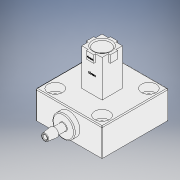
# Autodesk Inventor part: 9mm_ball_holder
Saved by Autodesk Inventor 2019 (Build 230136000, 136)
## iProperties
Created: 2019-03-11
Part Number: 9mm_ball_holder
Material: ABS Plastic
Document SubType Name: Modeling
Designer: Wilson Lab
Density: 1.06 g/cm^3
Appearance: Smooth - White
Author: Wilson Lab
Autodesk Inventor part; units mm, degrees
ref_plane "YZ Plane" through (0, 0, 0) normal (1, 0, 0) x (0, 1, 0)
ref_plane "XZ Plane" through (0, 0, 0) normal (0, 1, 0) x (-1, 0, 0)
ref_plane "XY Plane" through (0, 0, 0) normal (0, 0, 1) x (1, 0, 0)
sketch "Sketch1" plane through (0, 0, 0) normal (0, 0, 1) x (1, 0, 0)
  line L0 (0, 0) -> (-5.5, 0) construction
  line L1 (-5.5, 0) -> (-5.5, 20) construction
  line L2 (-5.5, 20) -> (0, 20) construction
  line L3 (0, 20) -> (0, 0) construction
  circle A0 centre (0, 20.35) radius 4.5 construction
  line L4 (-5.5, 20) -> (-5.1335, 20)
  line L5 (-0.75, 15.3188) -> (-0.75, 0)
  arc A1 (-4.4001, 19.4071) -> (-1.2857, 16.0376) centre (0, 20.35) ccw
  arc A2 (-0.75, 15.3188) -> (-1.2857, 16.0376) centre (-1.5, 15.3188) ccw
  arc A3 (-4.4001, 19.4071) -> (-5.1335, 20) centre (-5.1335, 19.25) ccw
  line L6 (-5.5, 20) -> (-5.5, 0)
  line L7 (-5.5, 0) -> (-0.75, 0)
  point P0 (-4.4864, 20)
  point P1 (-0.75, 15.9129)
  dimension "d1" = 20
  dimension "d5" = 9
  dimension "d6" = 0.35
  dimension "d7" = 0.75
  dimension "d8" = 0.75
  dimension "d9" = 0.75
  dimension "d133" = 5.5
  dimension "d134" = 1.0136
  constraints: 18 end point, 10 point on circle, 5 point on line, 4 centre point, 4 tangent, 3 perpendicular, 2 parallel, 1 collinear, 1 concentric, 1 horizontal
  measures "d1" distance between parallel lines of L0 L2
  measures "d5" diameter of A0
  measures "d6" distance of A0.centre L2.end
  measures "d7" distance between parallel lines of L3 L5
  measures "d8" radius of A2
  measures "d9" radius of A3
  measures "d133" distance between parallel lines of L1 L3
  measures "d134" distance of A0.start L1.end
revolve "Revolution1" add sketch "Sketch1" angle 360 about axis through (0, 20, 0) along (0, -1, 0)
ref_plane "Work Plane1" through (0, 20, 0) normal (0, 1, 0) x (1, 0, 0)
sketch "Sketch2" plane through (0, 20, 0) normal (0, 1, 0) x (1, 0, 0)
  circle A0 centre (0, 0) radius 5.5 projected
  circle A1 centre (0, 0) radius 5.5 construction
  line L0 (-5.5, -5.5) -> (5.5, -5.5)
  line L1 (5.5, -5.5) -> (5.5, 5.5)
  line L2 (5.5, 5.5) -> (-5.5, 5.5)
  line L3 (-5.5, 5.5) -> (-5.5, -5.5)
  circle A2 centre (0, 0) radius 1.2857 projected
  line L4 (-5.5, -5.5) -> (5.5, 5.5) construction
  line L5 (5.5, -5.5) -> (-5.5, 5.5) construction
  point P0 (0, 0)
  dimension "d124" = 0
  constraints: 12 end point, 2 midpoint, 2 parallel, 2 tangent, 1 centre point, 1 coincident, 1 horizontal, 1 perpendicular
  measures "d124" distance edge to line of A0 L1
extrude "Extrusion1" add sketch "Sketch2" against normal up to surface (20 mm away) contours L1 L0 A0 | A0 L2 L1 | A0 L3 L2 | L0 L3 A0
ref_plane "Work Plane7" through (0, 0, 0) normal (0, -1, 0) x (1, 0, 0)
sketch "Sketch11" plane through (0, 0, 0) normal (0, -1, 0) x (1, 0, 0)
  line L0 (0, 18) -> (0, 0) construction
  line L1 (-18, -18) -> (18, -18)
  line L2 (18, -18) -> (18, 18)
  line L3 (18, 18) -> (-18, 18)
  line L4 (-18, 18) -> (-18, -18)
  line L5 (-18, -18) -> (18, 18) construction
  line L6 (18, -18) -> (-18, 18) construction
  dimension "d60" = 36
  dimension "d61" = 36
  constraints: 14 end point, 3 midpoint, 2 parallel, 1 horizontal, 1 perpendicular
  measures "d60" distance of L1.end L2.end
  measures "d61" distance of L2.end L3.end
extrude "Extrusion6" add sketch "Sketch11" along normal blind 15
sketch "Sketch16" plane through (-18, 0, -18) normal (-1, 0, 0) x (0, 0, 1)
  line L0 (36, 0) -> (0, 0) construction
  line L1 (0, 0) -> (0, -15) construction
  line L2 (36, -15) -> (0, -15) construction
  line L3 (36, 0) -> (36, -15) construction
  line L4 (18.75, 15.3188) -> (18.75, 0) construction
  line L5 (17.25, 15.3188) -> (17.25, 0) construction
  line L6 (18, -7.5) -> (18, 0) construction
  line L7 (36, 0) -> (36, -15) construction
  line L8 (36, 0) -> (36, -7.5) construction
  line L9 (18, -7.5) -> (36, -7.5) construction
  circle A0 centre (18, -7.5) radius 4.225
  dimension "d64" = 8.45
  constraints: 6 end point, 1 centre point, 1 coincident, 1 horizontal, 1 midpoint, 1 vertical
  measures "d64" diameter of A0
extrude "Extrusion7" cut sketch "Sketch16" against normal blind 32.7
sketch "Sketch17" plane through (0, 0, 0) normal (0, -1, 0) x (1, 0, 0)
  circle A0 centre (0, 0) radius 0.75 projected
  point P0 (0, 0)
ref_plane "Work Plane8" through (-18, 0, 0) normal (0, 0, 1) x (1, 0, 0)
sketch "Sketch18" plane through (-18, 0, 0) normal (0, 0, 1) x (1, 0, 0)
  line L0 (18, 0) -> (18, -10.576)
  line L1 (0, -11.725) -> (32.7, -11.725) projected
  constraints: 2 end point, 1 vertical
sweep "Sweep3" cut profiles "Sketch17" path "Sketch18" path curves L0
fillet "Fillet1" radius 3 1 edges at (-0.75, -3.275, -0.001)
sketch "Sketch19" plane through (0, 0, 0) normal (0, 1, 0) x (1, 0, 0)
  line L0 (18, -18) -> (-18, -18) construction
  line L1 (18, 18) -> (18, -18) construction
  line L2 (-18, 18) -> (18, 18) construction
  line L3 (-18, -18) -> (-18, 18) construction
  line L4 (-12.7, 12.7) -> (12.7, 12.7) construction
  line L5 (12.7, 12.7) -> (12.7, -12.7) construction
  line L6 (12.7, -12.7) -> (-12.7, -12.7) construction
  line L7 (-12.7, -12.7) -> (-12.7, 12.7) construction
  circle A0 centre (0, 0) radius 1.2857 construction
  line L8 (-12.7, 12.7) -> (12.7, -12.7) construction
  line L9 (12.7, 12.7) -> (-12.7, -12.7) construction
  point P0 (0, 0)
  dimension "d70" = 25.4
  dimension "d71" = 25.4
  constraints: 12 end point, 4 coincident, 2 midpoint, 2 parallel, 1 horizontal, 1 perpendicular
  measures "d70" distance of L4.end L5.end
  measures "d71" distance of L5.end L6.end
hole "Hole3" at (12.7, 0, -12.7) at (12.7, 0, 12.7) at (-12.7, 0, 12.7) at (-12.7, 0, -12.7) direction (0, -1, 0) diameter 4.496 end through all counterbore diameter 7.938 counterbore depth 4.166
sketch "Sketch21" plane through (-18, 0, 0) normal (0, 0, 1) x (1, 0, 0)
  line L0 (0, -11.725) -> (0, -3.275) construction
  line L1 (0, 0) -> (0, -15) construction
  line L2 (0, -7.5) -> (-3, -7.5)
  line L3 (-3, -9.6296) -> (-3, -13.5)
  line L4 (-3, -13.5) -> (0, -13.5)
  line L5 (0, -13.5) -> (0, -7.5) construction
  line L6 (-3.25, -9.3796) -> (-8, -9.3796)
  arc A0 (-3, -9.6296) -> (-3.25, -9.3796) centre (-3.25, -9.6296) ccw
  line L7 (-8, -9.3796) -> (-8, -9.913)
  line L8 (-8, -9.913) -> (-12.8561, -9.4031)
  line L9 (-8, -9.3796) -> (-13.08, -9.3796) construction
  line L10 (-12.83, -8.65) -> (0, -8.65)
  line L11 (-13.08, -8.9) -> (-13.08, -9.1545)
  arc A1 (-12.83, -8.65) -> (-13.08, -8.9) centre (-12.83, -8.9) ccw
  arc A2 (-13.08, -9.1545) -> (-12.8561, -9.4031) centre (-12.83, -9.1545) ccw
  line L12 (0, -8.65) -> (0, -13.5)
  point P0 (18, 0)
  point P1 (-3, -9.3796)
  dimension "d79" = 3
  dimension "d80" = 6
  dimension "d81" = 5
  dimension "d82" = 1.8796
  dimension "d83" = 0.25
  dimension "d84" = 2.413
  dimension "d85" = 5.08
  dimension "d86" = 1.15
  dimension "d87" = 0.25
  dimension "d88" = 0.25
  constraints: 22 end point, 6 point on circle, 6 point on line, 6 tangent, 3 centre point, 3 horizontal, 2 parallel, 2 perpendicular, 2 vertical, 1 collinear, 1 midpoint
  measures "d79" distance of L3.end L4.end
  measures "d80" distance between parallel lines of L2 L4
  measures "d81" distance of point (-3, -9.38) L6.end
  measures "d82" distance between parallel lines of L2 L6
  measures "d83" radius of A0
  measures "d84" distance from line of L2 L7.end
  measures "d85" horizontal distance of L7.end L9.end
  measures "d86" distance between parallel lines of L10 L2
  measures "d87" radius of A1
  measures "d88" radius of A2
revolve "Revolution2" add sketch "Sketch21" angle 360 about axis through (-18, -7.5, 0) along (-1, 0, 0)
fillet "Fillet2" radius 0.5 9 edges at (-21, -1.5, 0) (0, 0, -18) (-18, 0, 0) (0, 0, 18) (18, 0, 0) (18, -7.5, 18) (-18, -7.5, 18) (-18, -7.5, -18) (18, -7.5, -18)
sketch "Sketch28" plane through (-5.5, 20, -5.5) normal (-1, 0, 0) x (0, 0, 1)
  line L0 (0, -20) -> (11, -20) construction
  line L1 (11, 0) -> (11, -20) construction
  line L2 (0, 0) -> (11, 0) construction
  line L3 (0, 0) -> (0, -20) construction
  line L4 (3.5, -4) -> (7.5, -4)
  line L5 (7.5, -4) -> (7.5, 0)
  line L6 (7.5, 0) -> (3.5, 0)
  line L7 (3.5, 0) -> (3.5, -4)
  line L8 (3.5, -2) -> (0, -2) construction
  line L9 (7.5, -2) -> (11, -2) construction
  point P0 (5.5, -20)
  dimension "d125" = 0
  dimension "d126" = 4
  constraints: 12 end point, 3 point on line, 2 equal length, 2 midpoint, 2 parallel, 2 perpendicular, 1 horizontal
  measures "d125" distance between parallel lines of L2 L6
  measures "d126" distance of L4.end L5.end
extrude "Extrusion13" add sketch "Sketch28" along normal blind 1
pattern_circular "Circular Pattern1" count 4 over 360 about axis through (0, -10, 0) along (0, 1, 0) of "Extrusion13"
sketch "Sketch29" plane through (-5.5, 0, -5.5) normal (-1, 0, 0) x (0, 0, 1)
  line L0 (0, 20) -> (0, 0) construction
  line L1 (0, 10) -> (11, 10) construction
  line L2 (11, 20) -> (11, 0) construction
  line L3 (0, 10) -> (11, 10) construction
  line L4 (11, 10) -> (11, 8) construction
  line L5 (11, 8) -> (0, 8) construction
  line L6 (0, 8) -> (0, 10) construction
  line L7 (0, 9) -> (11, 9) construction
  line L8 (11, 20) -> (11, 0) construction
  line L9 (0, 10) -> (0, 9) construction
  line L10 (11, 10) -> (11, 9) construction
  spline S0 degree 2 poles (4.1469, 9.0742) (4.1469, 9.0526) (4.1423, 9.0225) (4.1338, 9.0047) (4.1235, 8.9972) (4.116, 8.9972) knots 0 0 0 1 2 3 4 4 4
  line L11 (4.116, 8.9972) -> (3.5667, 8.9972)
  spline S1 degree 2 poles (3.5667, 8.9972) (3.5601, 8.9972) (3.5498, 9.0047) (3.5413, 9.0225) (3.5366, 9.0526) (3.5366, 9.0742) knots 0 0 0 1 2 3 4 4 4
  spline S2 degree 2 poles (3.5366, 9.0742) (3.5366, 9.0958) (3.5404, 9.1258) (3.5488, 9.1446) (3.5601, 9.1531) (3.5667, 9.1531) knots 0 0 0 1 2 3 4 4 4
  line L12 (3.5667, 9.1531) -> (3.7516, 9.1531)
  line L13 (3.7516, 9.1531) -> (3.7516, 9.8019)
  line L14 (3.7516, 9.8019) -> (3.5911, 9.7136)
  spline S3 degree 2 poles (3.5911, 9.7136) (3.5742, 9.7052) (3.5516, 9.7014) (3.5385, 9.7146) (3.5338, 9.7465) (3.5338, 9.7756) knots 0 0 0 1 2 3 4 4 4
  spline S4 degree 2 poles (3.5338, 9.7756) (3.5338, 9.7944) (3.5357, 9.8178) (3.5413, 9.8347) (3.5526, 9.846) (3.562, 9.8516) knots 0 0 0 1 2 3 4 4 4
  line L15 (3.562, 9.8516) -> (3.7751, 9.9897)
  spline S5 degree 2 poles (3.7751, 9.9897) (3.7798, 9.9934) (3.7911, 9.9972) (3.8099, 9.9991) (3.8399, 10) (3.8634, 10) knots 0 0 0 1 2 3 4 4 4
  spline S6 degree 2 poles (3.8634, 10) (3.8925, 10) (3.9291, 9.9981) (3.9469, 9.9925) (3.9535, 9.9831) (3.9535, 9.9765) knots 0 0 0 1 2 3 4 4 4
  line L16 (3.9535, 9.9765) -> (3.9535, 9.1531)
  line L17 (3.9535, 9.1531) -> (4.116, 9.1531)
  spline S7 degree 2 poles (4.116, 9.1531) (4.1235, 9.1531) (4.1347, 9.1446) (4.1432, 9.1258) (4.1469, 9.0958) (4.1469, 9.0742) knots 0 0 0 1 2 3 4 4 4
  spline S8 degree 2 poles (4.9451, 9.0742) (4.9451, 9.0526) (4.9404, 9.0225) (4.9319, 9.0047) (4.9216, 8.9972) (4.9141, 8.9972) knots 0 0 0 1 2 3 4 4 4
  line L18 (4.9141, 8.9972) -> (4.3648, 8.9972)
  spline S9 degree 2 poles (4.3648, 8.9972) (4.3582, 8.9972) (4.3479, 9.0047) (4.3394, 9.0225) (4.3347, 9.0526) (4.3347, 9.0742) knots 0 0 0 1 2 3 4 4 4
  spline S10 degree 2 poles (4.3347, 9.0742) (4.3347, 9.0958) (4.3385, 9.1258) (4.3469, 9.1446) (4.3582, 9.1531) (4.3648, 9.1531) knots 0 0 0 1 2 3 4 4 4
  line L19 (4.3648, 9.1531) -> (4.5498, 9.1531)
  line L20 (4.5498, 9.1531) -> (4.5498, 9.8019)
  line L21 (4.5498, 9.8019) -> (4.3892, 9.7136)
  spline S11 degree 2 poles (4.3892, 9.7136) (4.3723, 9.7052) (4.3498, 9.7014) (4.3366, 9.7146) (4.3319, 9.7465) (4.3319, 9.7756) knots 0 0 0 1 2 3 4 4 4
  spline S12 degree 2 poles (4.3319, 9.7756) (4.3319, 9.7944) (4.3338, 9.8178) (4.3394, 9.8347) (4.3507, 9.846) (4.3601, 9.8516) knots 0 0 0 1 2 3 4 4 4
  line L22 (4.3601, 9.8516) -> (4.5732, 9.9897)
  spline S13 degree 2 poles (4.5732, 9.9897) (4.5779, 9.9934) (4.5892, 9.9972) (4.608, 9.9991) (4.638, 10) (4.6615, 10) knots 0 0 0 1 2 3 4 4 4
  spline S14 degree 2 poles (4.6615, 10) (4.6906, 10) (4.7272, 9.9981) (4.7451, 9.9925) (4.7516, 9.9831) (4.7516, 9.9765) knots 0 0 0 1 2 3 4 4 4
  line L23 (4.7516, 9.9765) -> (4.7516, 9.1531)
  line L24 (4.7516, 9.1531) -> (4.9141, 9.1531)
  spline S15 degree 2 poles (4.9141, 9.1531) (4.9216, 9.1531) (4.9329, 9.1446) (4.9413, 9.1258) (4.9451, 9.0958) (4.9451, 9.0742) knots 0 0 0 1 2 3 4 4 4
  spline S16 degree 2 poles (6.2052, 9.0235) (6.2052, 9.016) (6.1958, 9.0038) (6.1742, 8.9962) (6.1376, 8.9925) (6.1085, 8.9925) knots 0 0 0 1 2 3 4 4 4
  spline S17 degree 2 poles (6.1085, 8.9925) (6.0793, 8.9925) (6.0427, 8.9962) (6.0202, 9.0038) (6.0117, 9.016) (6.0117, 9.0235) knots 0 0 0 1 2 3 4 4 4
  line L25 (6.0117, 9.0235) -> (6.0117, 9.43)
  spline S18 degree 2 poles (6.0117, 9.43) (6.0117, 9.4648) (5.9986, 9.5221) (5.9723, 9.5624) (5.931, 9.585) (5.9028, 9.585) knots 0 0 0 1 2 3 4 4 4
  spline S19 degree 2 poles (5.9028, 9.585) (5.8681, 9.585) (5.7977, 9.5315) (5.7563, 9.4798) knots 0 0 0 1 2 2 2
  line L26 (5.7563, 9.4798) -> (5.7563, 9.0235)
  spline S20 degree 2 poles (5.7563, 9.0235) (5.7563, 9.016) (5.7469, 9.0038) (5.7244, 8.9962) (5.6878, 8.9925) (5.6596, 8.9925) knots 0 0 0 1 2 3 4 4 4
  spline S21 degree 2 poles (5.6596, 8.9925) (5.6315, 8.9925) (5.5948, 8.9962) (5.5723, 9.0038) (5.5629, 9.016) (5.5629, 9.0235) knots 0 0 0 1 2 3 4 4 4
  line L27 (5.5629, 9.0235) -> (5.5629, 9.43)
  spline S22 degree 2 poles (5.5629, 9.43) (5.5629, 9.4648) (5.5498, 9.5221) (5.5235, 9.5624) (5.4822, 9.585) (5.454, 9.585) knots 0 0 0 1 2 3 4 4 4
  spline S23 degree 2 poles (5.454, 9.585) (5.4183, 9.585) (5.3479, 9.5315) (5.3066, 9.4798) knots 0 0 0 1 2 2 2
  line L28 (5.3066, 9.4798) -> (5.3066, 9.0235)
  spline S24 degree 2 poles (5.3066, 9.0235) (5.3066, 9.016) (5.2972, 9.0038) (5.2746, 8.9962) (5.238, 8.9925) (5.2099, 8.9925) knots 0 0 0 1 2 3 4 4 4
  spline S25 degree 2 poles (5.2099, 8.9925) (5.1817, 8.9925) (5.1451, 8.9962) (5.1225, 9.0038) (5.1131, 9.016) (5.1131, 9.0235) knots 0 0 0 1 2 3 4 4 4
  line L29 (5.1131, 9.0235) -> (5.1131, 9.7089)
  spline S26 degree 2 poles (5.1131, 9.7089) (5.1131, 9.7164) (5.1207, 9.7286) (5.1404, 9.7362) (5.1723, 9.7399) (5.1958, 9.7399) knots 0 0 0 1 2 3 4 4 4
  spline S27 degree 2 poles (5.1958, 9.7399) (5.2202, 9.7399) (5.2531, 9.7362) (5.2709, 9.7286) (5.2784, 9.7164) (5.2784, 9.7089) knots 0 0 0 1 2 3 4 4 4
  line L30 (5.2784, 9.7089) -> (5.2784, 9.63)
  spline S28 degree 2 poles (5.2784, 9.63) (5.3357, 9.6911) (5.4484, 9.7531) (5.5103, 9.7531) knots 0 0 0 1 2 2 2
  spline S29 degree 2 poles (5.5103, 9.7531) (5.5526, 9.7531) (5.6202, 9.7352) (5.6737, 9.7023) (5.7122, 9.6563) (5.7254, 9.6272) knots 0 0 0 1 2 3 4 4 4
  spline S30 degree 2 poles (5.7254, 9.6272) (5.7563, 9.661) (5.8155, 9.708) (5.8728, 9.738) (5.931, 9.7531) (5.961, 9.7531) knots 0 0 0 1 2 3 4 4 4
  spline S31 degree 2 poles (5.961, 9.7531) (6.0296, 9.7531) (6.1225, 9.707) (6.1808, 9.6282) (6.2052, 9.5211) (6.2052, 9.462) knots 0 0 0 1 2 3 4 4 4
  line L31 (6.2052, 9.462) -> (6.2052, 9.0235)
  spline S32 degree 2 poles (7.4869, 9.0235) (7.4869, 9.016) (7.4775, 9.0038) (7.4559, 8.9962) (7.4192, 8.9925) (7.3901, 8.9925) knots 0 0 0 1 2 3 4 4 4
  spline S33 degree 2 poles (7.3901, 8.9925) (7.361, 8.9925) (7.3244, 8.9962) (7.3019, 9.0038) (7.2934, 9.016) (7.2934, 9.0235) knots 0 0 0 1 2 3 4 4 4
  line L32 (7.2934, 9.0235) -> (7.2934, 9.43)
  spline S34 degree 2 poles (7.2934, 9.43) (7.2934, 9.4648) (7.2803, 9.5221) (7.254, 9.5624) (7.2127, 9.585) (7.1845, 9.585) knots 0 0 0 1 2 3 4 4 4
  spline S35 degree 2 poles (7.1845, 9.585) (7.1498, 9.585) (7.0793, 9.5315) (7.038, 9.4798) knots 0 0 0 1 2 2 2
  line L33 (7.038, 9.4798) -> (7.038, 9.0235)
  spline S36 degree 2 poles (7.038, 9.0235) (7.038, 9.016) (7.0286, 9.0038) (7.0061, 8.9962) (6.9695, 8.9925) (6.9413, 8.9925) knots 0 0 0 1 2 3 4 4 4
  spline S37 degree 2 poles (6.9413, 8.9925) (6.9131, 8.9925) (6.8765, 8.9962) (6.854, 9.0038) (6.8446, 9.016) (6.8446, 9.0235) knots 0 0 0 1 2 3 4 4 4
  line L34 (6.8446, 9.0235) -> (6.8446, 9.43)
  spline S38 degree 2 poles (6.8446, 9.43) (6.8446, 9.4648) (6.8315, 9.5221) (6.8052, 9.5624) (6.7638, 9.585) (6.7357, 9.585) knots 0 0 0 1 2 3 4 4 4
  spline S39 degree 2 poles (6.7357, 9.585) (6.7, 9.585) (6.6296, 9.5315) (6.5883, 9.4798) knots 0 0 0 1 2 2 2
  line L35 (6.5883, 9.4798) -> (6.5883, 9.0235)
  spline S40 degree 2 poles (6.5883, 9.0235) (6.5883, 9.016) (6.5789, 9.0038) (6.5563, 8.9962) (6.5197, 8.9925) (6.4915, 8.9925) knots 0 0 0 1 2 3 4 4 4
  spline S41 degree 2 poles (6.4915, 8.9925) (6.4634, 8.9925) (6.4268, 8.9962) (6.4042, 9.0038) (6.3948, 9.016) (6.3948, 9.0235) knots 0 0 0 1 2 3 4 4 4
  line L36 (6.3948, 9.0235) -> (6.3948, 9.7089)
  spline S42 degree 2 poles (6.3948, 9.7089) (6.3948, 9.7164) (6.4023, 9.7286) (6.4221, 9.7362) (6.454, 9.7399) (6.4775, 9.7399) knots 0 0 0 1 2 3 4 4 4
  spline S43 degree 2 poles (6.4775, 9.7399) (6.5019, 9.7399) (6.5347, 9.7362) (6.5526, 9.7286) (6.5601, 9.7164) (6.5601, 9.7089) knots 0 0 0 1 2 3 4 4 4
  line L37 (6.5601, 9.7089) -> (6.5601, 9.63)
  spline S44 degree 2 poles (6.5601, 9.63) (6.6174, 9.6911) (6.73, 9.7531) (6.792, 9.7531) knots 0 0 0 1 2 2 2
  spline S45 degree 2 poles (6.792, 9.7531) (6.8343, 9.7531) (6.9019, 9.7352) (6.9554, 9.7023) (6.9939, 9.6563) (7.007, 9.6272) knots 0 0 0 1 2 3 4 4 4
  spline S46 degree 2 poles (7.007, 9.6272) (7.038, 9.661) (7.0972, 9.708) (7.1545, 9.738) (7.2127, 9.7531) (7.2427, 9.7531) knots 0 0 0 1 2 3 4 4 4
  spline S47 degree 2 poles (7.2427, 9.7531) (7.3113, 9.7531) (7.4042, 9.707) (7.4624, 9.6282) (7.4869, 9.5211) (7.4869, 9.462) knots 0 0 0 1 2 3 4 4 4
  line L38 (7.4869, 9.462) -> (7.4869, 9.0235)
  point P0 (5.5, 0)
  dimension "d139" = 1
  constraints: 8 end point, 5 midpoint, 2 coincident, 2 collinear, 1 horizontal, 1 point on line, 2 other
  measures "d139" distance between parallel lines of L7 L1
sketch "Sketch30" plane through (-6.5, 20, -5.5) normal (-1, 0, 0) x (0, 0, 1)
  line L0 (3.5, 0) -> (3.5, -4) construction
  line L1 (3.5, -2) -> (7.5, -2) construction
  line L2 (7.5, 0) -> (7.5, -4) construction
  line L3 (3.5, -2) -> (7.5, -2) construction
  line L4 (7.5, -2) -> (7.5, -5.2981) construction
  line L5 (7.5, -5.2981) -> (3.5, -5.2981) construction
  line L6 (3.5, -5.2981) -> (3.5, -2) construction
  line L7 (7.5, -4) -> (7.5, 0) projected
  spline S0 degree 2 poles (4.5864, -2.7146) (4.5864, -2.754) (4.5704, -2.7944) (4.5563, -2.7944) knots 0 0 0 1 2 2 2
  line L8 (4.5563, -2.7944) -> (4.4681, -2.7944)
  line L9 (4.4681, -2.7944) -> (4.4681, -2.9737)
  spline S1 degree 2 poles (4.4681, -2.9737) (4.4681, -2.9812) (4.4587, -2.9934) (4.4362, -3.0009) (4.3986, -3.0047) (4.3695, -3.0047) knots 0 0 0 1 2 3 4 4 4
  spline S2 degree 2 poles (4.3695, -3.0047) (4.3423, -3.0047) (4.3047, -3.0009) (4.2822, -2.9934) (4.2737, -2.9812) (4.2737, -2.9737) knots 0 0 0 1 2 3 4 4 4
  line L10 (4.2737, -2.9737) -> (4.2737, -2.7944)
  line L11 (4.2737, -2.7944) -> (3.8925, -2.7944)
  spline S3 degree 2 poles (3.8925, -2.7944) (3.8812, -2.7944) (3.8643, -2.7887) (3.8531, -2.77) (3.8474, -2.7333) (3.8474, -2.7033) knots 0 0 0 1 2 3 4 4 4
  spline S4 degree 2 poles (3.8474, -2.7033) (3.8474, -2.6789) (3.8493, -2.6432) (3.8549, -2.6131) (3.8653, -2.5878) (3.8728, -2.5728) knots 0 0 0 1 2 3 4 4 4
  line L12 (3.8728, -2.5728) -> (4.1826, -2.0272)
  spline S5 degree 2 poles (4.1826, -2.0272) (4.1864, -2.0197) (4.2052, -2.0103) (4.238, -2.0028) (4.2887, -2) (4.3254, -2) knots 0 0 0 1 2 3 4 4 4
  spline S6 degree 2 poles (4.3254, -2) (4.3648, -2) (4.4192, -2.0038) (4.4531, -2.0122) (4.4681, -2.0244) (4.4681, -2.0329) knots 0 0 0 1 2 3 4 4 4
  line L13 (4.4681, -2.0329) -> (4.4681, -2.6329)
  line L14 (4.4681, -2.6329) -> (4.5563, -2.6329)
  spline S7 degree 2 poles (4.5563, -2.6329) (4.5685, -2.6329) (4.5864, -2.6704) (4.5864, -2.7146) knots 0 0 0 1 2 2 2
  line L15 (4.2737, -2.1746) -> (4.2718, -2.1746)
  line L16 (4.2718, -2.1746) -> (4.0089, -2.6329)
  line L17 (4.0089, -2.6329) -> (4.2737, -2.6329)
  line L18 (4.2737, -2.6329) -> (4.2737, -2.1746)
  spline S8 degree 2 poles (5.8061, -2.9737) (5.8061, -2.9812) (5.7967, -2.9934) (5.7751, -3.0009) (5.7385, -3.0047) (5.7094, -3.0047) knots 0 0 0 1 2 3 4 4 4
  spline S9 degree 2 poles (5.7094, -3.0047) (5.6803, -3.0047) (5.6437, -3.0009) (5.6211, -2.9934) (5.6127, -2.9812) (5.6127, -2.9737) knots 0 0 0 1 2 3 4 4 4
  line L19 (5.6127, -2.9737) -> (5.6127, -2.5671)
  spline S10 degree 2 poles (5.6127, -2.5671) (5.6127, -2.5324) (5.5995, -2.4751) (5.5732, -2.4347) (5.5319, -2.4122) (5.5038, -2.4122) knots 0 0 0 1 2 3 4 4 4
  spline S11 degree 2 poles (5.5038, -2.4122) (5.469, -2.4122) (5.3986, -2.4657) (5.3573, -2.5174) knots 0 0 0 1 2 2 2
  line L20 (5.3573, -2.5174) -> (5.3573, -2.9737)
  spline S12 degree 2 poles (5.3573, -2.9737) (5.3573, -2.9812) (5.3479, -2.9934) (5.3254, -3.0009) (5.2887, -3.0047) (5.2606, -3.0047) knots 0 0 0 1 2 3 4 4 4
  spline S13 degree 2 poles (5.2606, -3.0047) (5.2324, -3.0047) (5.1958, -3.0009) (5.1732, -2.9934) (5.1638, -2.9812) (5.1638, -2.9737) knots 0 0 0 1 2 3 4 4 4
  line L21 (5.1638, -2.9737) -> (5.1638, -2.5671)
  spline S14 degree 2 poles (5.1638, -2.5671) (5.1638, -2.5324) (5.1507, -2.4751) (5.1244, -2.4347) (5.0831, -2.4122) (5.0549, -2.4122) knots 0 0 0 1 2 3 4 4 4
  spline S15 degree 2 poles (5.0549, -2.4122) (5.0192, -2.4122) (4.9488, -2.4657) (4.9075, -2.5174) knots 0 0 0 1 2 2 2
  line L22 (4.9075, -2.5174) -> (4.9075, -2.9737)
  spline S16 degree 2 poles (4.9075, -2.9737) (4.9075, -2.9812) (4.8981, -2.9934) (4.8756, -3.0009) (4.839, -3.0047) (4.8108, -3.0047) knots 0 0 0 1 2 3 4 4 4
  spline S17 degree 2 poles (4.8108, -3.0047) (4.7826, -3.0047) (4.746, -3.0009) (4.7235, -2.9934) (4.7141, -2.9812) (4.7141, -2.9737) knots 0 0 0 1 2 3 4 4 4
  line L23 (4.7141, -2.9737) -> (4.7141, -2.2883)
  spline S18 degree 2 poles (4.7141, -2.2883) (4.7141, -2.2808) (4.7216, -2.2685) (4.7413, -2.261) (4.7732, -2.2573) (4.7967, -2.2573) knots 0 0 0 1 2 3 4 4 4
  spline S19 degree 2 poles (4.7967, -2.2573) (4.8211, -2.2573) (4.854, -2.261) (4.8718, -2.2685) (4.8793, -2.2808) (4.8793, -2.2883) knots 0 0 0 1 2 3 4 4 4
  line L24 (4.8793, -2.2883) -> (4.8793, -2.3671)
  spline S20 degree 2 poles (4.8793, -2.3671) (4.9366, -2.3061) (5.0493, -2.2441) (5.1113, -2.2441) knots 0 0 0 1 2 2 2
  spline S21 degree 2 poles (5.1113, -2.2441) (5.1535, -2.2441) (5.2211, -2.262) (5.2746, -2.2948) (5.3131, -2.3408) (5.3263, -2.37) knots 0 0 0 1 2 3 4 4 4
  spline S22 degree 2 poles (5.3263, -2.37) (5.3573, -2.3362) (5.4164, -2.2892) (5.4737, -2.2592) (5.5319, -2.2441) (5.562, -2.2441) knots 0 0 0 1 2 3 4 4 4
  spline S23 degree 2 poles (5.562, -2.2441) (5.6305, -2.2441) (5.7235, -2.2901) (5.7817, -2.369) (5.8061, -2.4761) (5.8061, -2.5352) knots 0 0 0 1 2 3 4 4 4
  line L25 (5.8061, -2.5352) -> (5.8061, -2.9737)
  spline S24 degree 2 poles (7.0878, -2.9737) (7.0878, -2.9812) (7.0784, -2.9934) (7.0568, -3.0009) (7.0202, -3.0047) (6.9911, -3.0047) knots 0 0 0 1 2 3 4 4 4
  spline S25 degree 2 poles (6.9911, -3.0047) (6.962, -3.0047) (6.9254, -3.0009) (6.9028, -2.9934) (6.8944, -2.9812) (6.8944, -2.9737) knots 0 0 0 1 2 3 4 4 4
  line L26 (6.8944, -2.9737) -> (6.8944, -2.5671)
  spline S26 degree 2 poles (6.8944, -2.5671) (6.8944, -2.5324) (6.8812, -2.4751) (6.8549, -2.4347) (6.8136, -2.4122) (6.7854, -2.4122) knots 0 0 0 1 2 3 4 4 4
  spline S27 degree 2 poles (6.7854, -2.4122) (6.7507, -2.4122) (6.6803, -2.4657) (6.639, -2.5174) knots 0 0 0 1 2 2 2
  line L27 (6.639, -2.5174) -> (6.639, -2.9737)
  spline S28 degree 2 poles (6.639, -2.9737) (6.639, -2.9812) (6.6296, -2.9934) (6.607, -3.0009) (6.5704, -3.0047) (6.5423, -3.0047) knots 0 0 0 1 2 3 4 4 4
  spline S29 degree 2 poles (6.5423, -3.0047) (6.5141, -3.0047) (6.4775, -3.0009) (6.4549, -2.9934) (6.4455, -2.9812) (6.4455, -2.9737) knots 0 0 0 1 2 3 4 4 4
  line L28 (6.4455, -2.9737) -> (6.4455, -2.5671)
  spline S30 degree 2 poles (6.4455, -2.5671) (6.4455, -2.5324) (6.4324, -2.4751) (6.4061, -2.4347) (6.3648, -2.4122) (6.3366, -2.4122) knots 0 0 0 1 2 3 4 4 4
  spline S31 degree 2 poles (6.3366, -2.4122) (6.3009, -2.4122) (6.2305, -2.4657) (6.1892, -2.5174) knots 0 0 0 1 2 2 2
  line L29 (6.1892, -2.5174) -> (6.1892, -2.9737)
  spline S32 degree 2 poles (6.1892, -2.9737) (6.1892, -2.9812) (6.1798, -2.9934) (6.1573, -3.0009) (6.1207, -3.0047) (6.0925, -3.0047) knots 0 0 0 1 2 3 4 4 4
  spline S33 degree 2 poles (6.0925, -3.0047) (6.0643, -3.0047) (6.0277, -3.0009) (6.0052, -2.9934) (5.9958, -2.9812) (5.9958, -2.9737) knots 0 0 0 1 2 3 4 4 4
  line L30 (5.9958, -2.9737) -> (5.9958, -2.2883)
  spline S34 degree 2 poles (5.9958, -2.2883) (5.9958, -2.2808) (6.0033, -2.2685) (6.023, -2.261) (6.0549, -2.2573) (6.0784, -2.2573) knots 0 0 0 1 2 3 4 4 4
  spline S35 degree 2 poles (6.0784, -2.2573) (6.1028, -2.2573) (6.1357, -2.261) (6.1535, -2.2685) (6.161, -2.2808) (6.161, -2.2883) knots 0 0 0 1 2 3 4 4 4
  line L31 (6.161, -2.2883) -> (6.161, -2.3671)
  spline S36 degree 2 poles (6.161, -2.3671) (6.2183, -2.3061) (6.331, -2.2441) (6.393, -2.2441) knots 0 0 0 1 2 2 2
  spline S37 degree 2 poles (6.393, -2.2441) (6.4352, -2.2441) (6.5028, -2.262) (6.5563, -2.2948) (6.5948, -2.3408) (6.608, -2.37) knots 0 0 0 1 2 3 4 4 4
  spline S38 degree 2 poles (6.608, -2.37) (6.639, -2.3362) (6.6981, -2.2892) (6.7554, -2.2592) (6.8136, -2.2441) (6.8437, -2.2441) knots 0 0 0 1 2 3 4 4 4
  spline S39 degree 2 poles (6.8437, -2.2441) (6.9122, -2.2441) (7.0052, -2.2901) (7.0634, -2.369) (7.0878, -2.4761) (7.0878, -2.5352) knots 0 0 0 1 2 3 4 4 4
  line L32 (7.0878, -2.5352) -> (7.0878, -2.9737)
  point P0 (5.5, -20)
  constraints: 4 midpoint, 2 coincident, 2 end point, 2 other
extrude "Extrusion14" cut sketch "Sketch29" against normal blind 0.5
extrude "Extrusion15" cut sketch "Sketch30" against normal blind 0.5
body "Solid1"
